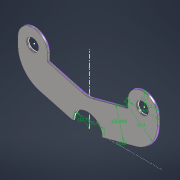
# Autodesk Inventor part: FixaçãoTanque_1
Saved by Autodesk Inventor 2022 (Build 260153000, 153)
## iProperties
Created: 2022-05-19
Part Number: FixaçãoTanque_1
Material: Liga de aço
Document SubType Name: Modeling
Designer: Gugarauj07
Density: 7.73 g/cm^3
Appearance: Semipolido
Author: Gugarauj07
Autodesk Inventor part; units mm, degrees
ref_plane "YZ Plane" through (0, 0, 0) normal (1, 0, 0) x (0, 1, 0)
ref_plane "XZ Plane" through (0, 0, 0) normal (0, 1, 0) x (-1, 0, 0)
ref_plane "XY Plane" through (0, 0, 0) normal (0, 0, 1) x (1, 0, 0)
sketch "Esboço1" plane through (0, 0, 0) normal (0, 0, 1) x (1, 0, 0)
  arc A0 (0, 12.7) -> (-12.7, 0) centre (0, 0) ccw
  circle A1 centre (-47.371, 39.2) radius 5.08
  line L0 (0, 0) -> (0, 58.6538)
  arc A2 (12.7, 0) -> (0, 12.7) centre (0, 0) ccw
  circle A3 centre (47.371, 39.2) radius 5.08
  line L1 (12.7, 0) -> (41.5415, 7.7281)
  line L2 (12.7, 0) -> (62.7, 0) construction
  line L3 (60.071, 39.2) -> (60.071, 31.8762)
  arc A4 (60.071, 39.2) -> (34.671, 39.2) centre (47.371, 39.2) ccw
  line L4 (-12.7, 0) -> (-41.5415, 7.7281)
  line L5 (-60.071, 39.2) -> (-60.071, 31.8762)
  arc A5 (-34.671, 39.2) -> (-60.071, 39.2) centre (-47.371, 39.2) ccw
  line L6 (34.671, 39.2) -> (34.671, 32.7)
  line L7 (34.671, 32.7) -> (4.8918, 24.7207)
  line L8 (-34.671, 39.2) -> (-34.671, 32.7)
  line L9 (-34.671, 32.7) -> (-4.8918, 24.7207)
  arc A6 (-4.8918, 24.7207) -> (4.8918, 24.7207) centre (0, 45.0927) ccw
  arc A7 (41.5415, 7.7281) -> (60.071, 31.8762) centre (34.6728, 32.1817) ccw
  arc A8 (-60.071, 31.8762) -> (-41.5415, 7.7281) centre (-34.6728, 32.1817) ccw
  point P0 (0, 25.2951)
  point P1 (0, 24.8739)
  dimension "d6" = 12.7
  dimension "d10" = 25.4
  dimension "d17" = 15
  dimension "d18" = 12.7
  dimension "d19" = 25.4
  dimension "d20" = 12.7
  dimension "d27" = 6.5
  dimension "d32" = 25.8993
  dimension "d33" = 25.4
  constraints: 20 end point, 14 point on circle, 10 symmetric about line, 9 centre point, 3 vertical, 2 point on line, 1 coincident, 1 horizontal, 1 parallel, 9 other
  measures "d6" radius of A0
  measures "d10" distance of L1.start L4.start
  measures "d17" angle of L2 L1
  measures "d18" distance of A3.centre L3.start
  measures "d19" distance of L3.start L6.start
  measures "d20" radius of A4
  measures "d27" distance of L6.start L6.end
  measures "d32" distance between parallel lines of L1 L7
  measures "d33" radius of A7
extrude "Extrusion2" add sketch "Esboço1" along normal blind 1.5
